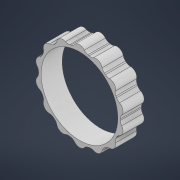
# Autodesk Inventor part: Wheel Outer
Saved by Autodesk Inventor 2022.1 (Build 261234000, 234)
## iProperties
Created: 2021-10-11
Part Number: Wheel Outer
Material: Generic
Document SubType Name: Modeling
Designer: Santiago Martínez
Mass: 12.0694 g
Surface Area: 87.9308 cm^2
Volume: 12.0694 cm^3
Density: 1 g/cm^3
Appearance: Default
Author: Santiago Martínez
Autodesk Inventor part; units mm, degrees
ref_plane "YZ Plane" through (0, 0, 0) normal (1, 0, 0) x (0, 1, 0)
ref_plane "XZ Plane" through (0, 0, 0) normal (0, 1, 0) x (-1, 0, 0)
ref_plane "XY Plane" through (0, 0, 0) normal (0, 0, 1) x (1, 0, 0)
sketch "Profile S" plane through (0, 0, 0) normal (0, 0, 1) x (1, 0, 0)
  circle A0 centre (0, 0) radius 32 projected
  circle A1 centre (0, 0) radius 31
  circle A2 centre (0, 0) radius 33
  dimension "d0" = 62
  dimension "d1" = 66
  constraints: 2 centre point, 2 coincident
  measures "d0" diameter of A1
  measures "d1" diameter of A2
extrude "Outer Wall" add sketch "Profile S" along normal blind 17 contours A0 | A2
sketch "Sketch3" plane through (0, 0, 17) normal (0, 0, 1) x (1, 0, 0)
  circle A0 centre (0, 0) radius 31 projected
  circle A1 centre (0, 0) radius 33 projected
  circle A2 centre (0, 0) radius 33 projected
  circle A3 centre (0, 0) radius 33 projected
  arc A4 (3.9319, 34.0887) -> (-3.9319, 34.0887) centre (0, 31) ccw
  arc A5 (-6.8291, 32.2857) -> (-3.9319, 34.0887) centre (-7.8638, 37.1774) ccw
  arc A6 (3.9319, 34.0887) -> (6.8291, 32.2857) centre (7.8638, 37.1774) ccw
  point P0 (6.8291, 32.2857)
  dimension "d20" = 31
  dimension "d21" = 10
  dimension "d22" = 5
  constraints: 8 point on circle, 4 tangent, 3 centre point, 2 horizontal alignment, 1 vertical alignment
  measures "d20" distance of point (0, 0) A4.centre
  measures "d21" diameter of A4
  measures "d22" radius of A5
extrude "Extrusion4" add sketch "Sketch3" against normal blind 17 contours A1 A5 A4 A6
pattern_circular "Circular Pattern3" count 14 over 360 about axis through (0, 0, 0) along (0, 0, 1) of "Extrusion4"
body "Solid1"
